Autodesk Fusion 360 part; units mm, degrees
note: some values were not read from the file. Chosen so that the rebuilt part matches the saved one: a direction. Set by a fixed rule: which sketch regions a step uses; which face or edge a step refers to.
(part 6 of 6)
sketch "Sketch34" plane through (0, 0, 0) normal (0, 1, 0) x (1, 0, 0)
  line L0 (0, 0) -> (0, -96.5685)
  line L1 (0, -96.5685) -> (160, -96.5685)
  line L2 (200, -56.5685) -> (200, 0)
  line L3 (200, 0) -> (196, 0)
  arc A0 (160, -96.5685) -> (200, -56.5685) centre (160, -56.5685) ccw
  line L4 (0, 0) -> (0, -88.5685)
  line L5 (0, -88.5685) -> (164, -88.5685)
  line L6 (196, -56.5685) -> (196, 4)
  arc A1 (164, -88.5685) -> (196, -56.5685) centre (164, -56.5685) ccw
  line L7 (196, -56.5685) -> (200, -56.5685)
  line L8 (0, -88.5685) -> (0, -96.5685)
  line L9 (0, 0) -> (0, -83.5685)
  line L10 (0, -83.5685) -> (164, -83.5685)
  line L11 (191, -56.5685) -> (191, -24.5685)
  arc A2 (164, -83.5685) -> (191, -56.5685) centre (164, -56.5685) ccw
  line L12 (0, 0) -> (0, -75.5685)
  line L13 (0, -75.5685) -> (168, -75.5685)
  line L14 (187, -56.5685) -> (187, 0)
  arc A3 (168, -75.5685) -> (187, -56.5685) centre (168, -56.5685) ccw
  line L15 (196, -56.5685) -> (196, -56.3185)
  line L16 (196, -56.5685) -> (196, -56.8185)
  line L17 (196, 0) -> (256, 0) construction
  line L18 (200, 0) -> (143.4315, -56.5685)
  line L19 (200, 0) -> (260, 0) construction
  line L20 (143.4315, -56.5685) -> (187, -56.5685)
  line L21 (187, -56.5685) -> (226.5075, -50.3112)
  line L22 (187, -56.5685) -> (217.0736, -56.5685) construction
  point P0 (200, -96.5685)
  point P1 (196, -88.5685)
  point P2 (191, -83.5685)
  point P3 (187, -75.5685)
  dimension "d479" = 96.5685
  dimension "d480" = 200
  dimension "d481" = 96.5685
  dimension "d482" = 4
  dimension "d483" = 40
  dimension "d484" = 88.5685
  dimension "d485" = 196
  dimension "d486" = 92.5685
  dimension "d487" = 32
  dimension "d488" = 83.5685
  dimension "d489" = 191
  dimension "d490" = 59
  dimension "d491" = 27
  dimension "d492" = 75.5685
  dimension "d493" = 187
  dimension "d494" = 75.5685
  dimension "d495" = 19
  dimension "d496" = 0.25
  dimension "d498" = 0.25
  dimension "d502" = 135
  dimension "d503" = 80
  dimension "d504" = 43.5685
  dimension "d505" = 40
  dimension "d506" = 9
  constraint coincident L0.start L4.start
  constraint vertical L0
  constraint perpendicular L0 L1
  constraint perpendicular L1 L2
  constraint perpendicular L2 L3
  constraint coincident P0 L1
  constraint coincident P0 L2
  constraint tangent L1 A0
  constraint tangent L2 A0
  constraint parallel L0 L4
  constraint perpendicular L4 L5
  constraint perpendicular L5 L6
  constraint coincident P1 L6
  constraint coincident P1 L5
  constraint tangent L6 A1
  constraint tangent L5 A1
  constraint perpendicular L5 L9
  constraint perpendicular L9 L10
  constraint perpendicular L10 L11
  constraint coincident P2 L10
  constraint coincident P2 L11
  constraint tangent L10 A2
  constraint tangent L11 A2
  constraint parallel L4 L12
  constraint perpendicular L12 L13
  constraint perpendicular L13 L14
  constraint coincident P3 L14
  constraint coincident P3 L13
  constraint tangent L14 A3
  constraint tangent L13 A3
  constraint perpendicular L7 L15
  constraint perpendicular L7 L16
  constraint horizontal L17
  constraint horizontal L19
  constraint horizontal L20
  constraint horizontal L22
  measures "d479" distance of L0.start L0.end
  measures "d480" distance of L0.end P0
  measures "d481" distance of P0 L2.end
  measures "d482" distance of L2.end L3.end
  measures "d483" radius of A0
  measures "d484" distance of L0.start L4.end
  measures "d485" distance of L4.end P1
  measures "d486" distance of P1 L6.end
  measures "d487" radius of A1
  measures "d488" distance of L0.start L9.end
  measures "d489" distance of L9.end P2
  measures "d490" distance of P2 L11.end
  measures "d491" radius of A2
  measures "d492" distance of L0.start L12.end
  measures "d493" distance of L12.end P3
  measures "d494" distance of P3 L14.end
  measures "d495" radius of A3
  measures "d496" distance of L6.start L15.end
  measures "d498" distance of L6.start L16.end
  measures "d502" angle of L18 L19
  measures "d503" distance of L2.end L18.end
  measures "d504" distance of L18.end L14.start
  measures "d505" distance of L14.start L21.end
  measures "d506" angle of L21 L22
extrude "Extrude51" add sketch "Sketch34" along normal blind 4 from surface at 4 separate body contours L0 L4 L9 L10 L11 A2 L13 A3 L21 | L0 L1 A0 L5 A1 L7 L8 L16 makes body 14 at (110.6667, 4, 78.2352) makes body 15 at (108, 4, 91.2352)
sketch "rail top 1" plane through (0, 8, 0) normal (0, 1, 0) x (-1, 0, 0)
  line L0 (-164, 88.5685) -> (0, 88.5685)
  line L1 (0, 88.5685) -> (0, 96.5685)
  line L2 (0, 96.5685) -> (-160, 96.5685)
  arc A0 (-160, 96.5685) -> (-200, 56.5685) centre (-160, 56.5685) ccw
  line L3 (-200, 56.5685) -> (-196, 56.5685)
  arc A1 (-164, 88.5685) -> (-196, 56.5685) centre (-164, 56.5685) ccw
  line L4 (0, 96.5685) -> (-8, 96.5685)
  line L5 (-8, 96.5685) -> (-8, 92.5685)
  line L6 (-10, 90.5685) -> (-6, 90.5685)
  line L7 (-6, 90.5685) -> (-6, 94.5685)
  line L8 (-6, 94.5685) -> (-10, 94.5685)
  line L9 (-10, 94.5685) -> (-10, 90.5685)
  line L10 (-10, 90.5685) -> (-6, 94.5685) construction
  line L11 (-6, 90.5685) -> (-10, 94.5685) construction
  point P0 (-8, 92.5685)
  dimension "d513" = 8
  dimension "d514" = 4
  dimension "d515" = 4
  dimension "d516" = 4
  constraint coincident L1.end L2.start
  constraint perpendicular L1 L4
  constraint perpendicular L4 L5
  constraint horizontal L6
  constraint perpendicular L6 L7
  constraint parallel L6 L8
  constraint parallel L7 L9
  constraint coincident L10 P0
  constraint coincident L11 P0
  constraint coincident P0 L5.end
  measures "d513" distance of L1.end L4.end
  measures "d514" distance of L4.end P0
  measures "d515" distance of L7.end L8.end
  measures "d516" distance of L6.end L7.end
extrude "Extrude53" cut sketch "rail top 1" against normal blind 8 contours L6 L7 L8 L9 bodies 2 15
pattern_linear "R-Pattern16" count 3 spacing 72 along (1, 0, 0) of "Extrude53"
sketch "rail bottom 1" plane through (0, 8, 0) normal (0, 1, 0) x (-1, 0, 0)
  line L0 (0, 75.5685) -> (0, 83.5685)
  line L1 (0, 83.5685) -> (-164, 83.5685)
  arc A0 (-164, 83.5685) -> (-191, 56.5685) centre (-164, 56.5685) ccw
  line L2 (-191, 55.935) -> (-187, 56.5685)
  arc A1 (-168, 75.5685) -> (-187, 56.5685) centre (-168, 56.5685) ccw
  line L3 (-168, 75.5685) -> (0, 75.5685)
  line L4 (0, 0) -> (0, 79.5685)
  line L5 (0, 79.5685) -> (-8, 79.5685)
  line L6 (-10, 77.5685) -> (-6, 77.5685)
  line L7 (-6, 77.5685) -> (-6, 81.5685)
  line L8 (-6, 81.5685) -> (-10, 81.5685)
  line L9 (-10, 81.5685) -> (-10, 77.5685)
  line L10 (-10, 77.5685) -> (-6, 81.5685) construction
  line L11 (-6, 77.5685) -> (-10, 81.5685) construction
  line L12 (-191, 56.5685) -> (-191, 55.935)
  point P0 (-8, 79.5685)
  dimension "d523" = 79.5685
  dimension "d524" = 8
  dimension "d525" = 4
  dimension "d526" = 4
  constraint coincident L4.start origin
  constraint midpoint L0 L4.end
  constraint perpendicular L0 L5
  constraint horizontal L6
  constraint perpendicular L6 L7
  constraint parallel L6 L8
  constraint parallel L7 L9
  constraint coincident L10 P0
  constraint coincident L11 P0
  constraint coincident P0 L5.end
  measures "d523" distance of L4.start L4.end
  measures "d524" distance of L4.end P0
  measures "d525" distance of L7.end L8.end
  measures "d526" distance of L6.end L7.end
extrude "Extrude54" cut sketch "rail bottom 1" against normal blind 8 contours L6 L7 L8 L9 bodies 2 14
pattern_linear "R-Pattern17" count 3 spacing 72 along (1, 0, 0) of "Extrude54"
sketch "fingur top rail" plane through (0, 0, 0) normal (-1, 0, 0) x (0, -1, 0)
  line L0 (-4, 88.5685) -> (-4, 96.5685)
  line L1 (-4, 96.5685) -> (-8, 96.5685)
  line L2 (-8, 96.5685) -> (-8, 88.5685)
  line L3 (-8, 88.5685) -> (-4, 88.5685)
  line L4 (-8, 96.5685) -> (-4, 96.5685)
  line L5 (-4, 96.5685) -> (-4, 93.9019)
  line L6 (-4, 93.9019) -> (-8, 93.9019)
  line L7 (-8, 93.9019) -> (-8, 96.5685)
  dimension "d533" = 2.6667
  constraint horizontal L4
  constraint vertical L5
  constraint horizontal L6
  constraint vertical L7
  constraint coincident L0 L5.end
  constraint coincident L1.end L2.start
  measures "d533" distance of L0.end L5.end
extrude "Extrude55" cut sketch "fingur top rail" against normal blind 4 contours L0 L1 L2 L4 L5 L6 L7 bodies 15
pattern_linear "R-Pattern18" count 2 spacing 5.3333 along (0, 0, -1) of "Extrude55"
sketch "fingur bottom rail " plane through (0, 0, 0) normal (-1, 0, 0) x (0, -1, 0)
  line L0 (-4, 75.5685) -> (-4, 83.5685)
  line L1 (-4, 83.5685) -> (-8, 83.5685)
  line L2 (-8, 83.5685) -> (-8, 75.5685)
  line L3 (-8, 75.5685) -> (-4, 75.5685)
  line L4 (-4, 83.5685) -> (-8, 83.5685)
  line L5 (-8, 83.5685) -> (-8, 80.9019)
  line L6 (-8, 80.9019) -> (-4, 80.9019)
  line L7 (-4, 80.9019) -> (-4, 83.5685)
  dimension "d540" = 2.6667
  constraint horizontal L4
  constraint vertical L5
  constraint horizontal L6
  constraint vertical L7
  constraint coincident L2 L5.end
  constraint coincident L0.end L1.start
  measures "d540" distance of L1.end L5.end
extrude "Extrude56" cut sketch "fingur bottom rail " against normal blind 4 contours L0 L1 L2 L4 L5 L6 L7 bodies 14
pattern_linear "R-Pattern19" count 2 spacing 5.3333 along (0, 0, -1) of "Extrude56"
extrude "Extrude52" add 2 faces at (162, 8, 78.9019) (159.3333, 8, 91.9019) along direction (0, -1, 0) blind 4 separate body start surface through (136, 96, 13) normal (0, -1, 0) on bodies 14 15 makes body 16 at (159.3333, 96, 91.9019) makes body 17 at (162, 96, 78.9019)
pattern_linear "R-Pattern20" count 2 spacing 92 along (0, 1, 0) of "Extrude53", "R-Pattern16", "Extrude54", "R-Pattern17"
extrude "Extrude57" cut sketch "rail bottom 1" along normal through all contours L6 L7 L8 L9 bodies 3
pattern_linear "R-Pattern21" count 3 spacing 72 along (1, 0, 0) of "Extrude57"
extrude "Extrude58" cut sketch "rail top 1" along normal through all contours L6 L7 L8 L9 bodies 3
pattern_linear "R-Pattern22" count 3 spacing 72 along (1, 0, 0) of "Extrude58"
sketch "flex sc" plane through (0, 0, 0) normal (0, 0, 1) x (1, 0, 0)
  line L0 (0, 0) -> (250, 0)
  line L1 (250, 0) -> (468.8319, 0)
  line L2 (468.8319, 0) -> (468.8319, 92)
  line L3 (468.8319, 92) -> (250, 92)
  line L4 (250, 92) -> (250, 0)
  dimension "d574" = 250
  dimension "d575" = 218.8319
  dimension "d576" = 92
  constraint coincident L0.start origin
  constraint horizontal L0
  constraint horizontal L1
  constraint vertical L2
  constraint horizontal L3
  constraint vertical L4
  measures "d574" distance of L0.start L0.end
  measures "d575" distance of L0.end L1.end
  measures "d576" distance of L0.end L3.end
extrude "Extrude60" add sketch "flex sc" along normal blind 4 separate body makes body 18
sketch "pinni sc" plane through (0, 0, 0) normal (0, 0, 1) x (1, 0, 0)
  line L0 (0, -20) -> (8, -20)
  line L1 (8, -20) -> (8, -24)
  line L2 (8, -24) -> (0, -24)
  line L3 (0, -24) -> (0, -20)
  dimension "d579" = 8
  dimension "d580" = 4
  constraint horizontal L0
  constraint vertical L1
  constraint horizontal L2
  constraint vertical L3
  measures "d579" distance of L0.start L0.end
  measures "d580" distance of L0.start L2.end
extrude "Extrude61" add sketch "pinni sc" along normal blind 4 separate body makes body 19
pattern_linear "R-Pattern23" count 14 spacing 9 along (1, 0, 0) of bodies 19 makes body 20 at (11.6667, -20, 2.6667) makes body 21 at (20.6667, -20, 2.6667) makes body 22 at (29.6667, -20, 2.6667) makes body 23 at (38.6667, -20, 2.6667) makes body 24 at (47.6667, -20, 2.6667) makes body 25 at (56.6667, -20, 2.6667) makes body 26 at (65.6667, -20, 2.6667) makes body 27 at (74.6667, -20, 2.6667) makes body 28 at (83.6667, -20, 2.6667) makes body 29 at (92.6667, -20, 2.6667) makes body 30 at (101.6667, -20, 2.6667) makes body 31 at (110.6667, -20, 2.6667) makes body 32 at (119.6667, -20, 2.6667)
combine "Combine13" operation cut target body 2 tool bodies 6 keep tools
combine "Combine14" operation cut target body 3 tool bodies 6 keep tools
combine "Combine15" operation cut target body 2 tool bodies 13 12 11 10 9 keep tools
combine "Combine16" operation cut target body 3 tool bodies 13 12 11 10 9 keep tools
combine "Combine17" operation cut target body 4 tool bodies 15 14 16 17 keep tools
sketch "Sketch43" plane through (0, 0, 4) normal (0, 0, 1) x (-1, 0, 0)
  line L0 (-250, -92) -> (-250, 0)
  line L1 (-250, 0) -> (-468.8319, 0)
  line L2 (-468.8319, 0) -> (-468.8319, -92)
  line L3 (-468.8319, -92) -> (-250, -92)
  line L4 (-250, 0) -> (-258, 0)
  line L5 (-258, 0) -> (-258, -92)
  line L6 (-258, -92) -> (-250, -92)
  line L7 (-250, -92) -> (-250, 0)
  line L8 (-250, 0) -> (-252, 0)
  line L9 (-252, 0) -> (-252, -92)
  line L10 (-252, -92) -> (-250, -92)
  line L11 (-250, -92) -> (-250, 0)
  line L12 (-250, 0) -> (-256, 0)
  line L13 (-256, 0) -> (-256, -92)
  line L14 (-256, -92) -> (-250, -92)
  line L15 (-250, -92) -> (-250, 0)
  line L16 (-252, -4) -> (-256, -4)
  line L17 (-256, -4) -> (-256, -88)
  line L18 (-256, -88) -> (-252, -88)
  line L19 (-252, -88) -> (-252, -4)
  dimension "d594" = 8
  dimension "d625" = 2
  dimension "d626" = 92
  dimension "d627" = 6
  dimension "d628" = 92
  dimension "d629" = 4
  dimension "d630" = 84
  constraint horizontal L4
  constraint vertical L5
  constraint horizontal L6
  constraint vertical L7
  constraint coincident L3 L5.end
  constraint coincident L0.end L1.start
  constraint horizontal L8
  constraint vertical L9
  constraint horizontal L10
  constraint vertical L11
  constraint horizontal L12
  constraint vertical L13
  constraint horizontal L14
  constraint vertical L15
  constraint horizontal L16
  constraint vertical L17
  constraint horizontal L18
  constraint vertical L19
  constraint coincident L13 L17.end
  constraint coincident L9 L16.start
  measures "d594" distance of L5 L7
  measures "d625" distance of L0.end L8.end
  measures "d626" distance of L0.end L0.start
  measures "d627" distance of L0.end L12.end
  measures "d628" distance of L0.end L0.start
  measures "d629" distance of L4 L16
  measures "d630" distance of L16 L18
extrude "Extrude63" add sketch "Sketch43" along normal blind 12 from surface at -4 separate body contours L9 L13 L16 L17 L18 L19 makes body 33
sketch "Sketch44" plane through (0, 0, 0) normal (0, 0, -1) x (1, 0, 0)
  line L0 (256, -88) -> (252, -88)
  line L1 (252, -88) -> (252, -81.3333)
  line L2 (252, -81.3333) -> (256, -81.3333)
  line L3 (256, -81.3333) -> (256, -88)
  line L4 (252, -4) -> (252, -88)
  line L5 (252, -88) -> (256, -88)
  line L6 (256, -88) -> (256, -4)
  line L7 (256, -4) -> (252, -4)
  dimension "d613" = 6.6667
  constraint horizontal L0
  constraint vertical L1
  constraint horizontal L2
  constraint vertical L3
  measures "d613" distance of L0 L2
sketch "Sketch45" plane through (0, 0, 4) normal (0, 0, 1) x (-1, 0, 0)
  line L0 (-250, -92) -> (-250, 0)
  line L1 (-250, 0) -> (-468.8319, 0)
  line L2 (-468.8319, 0) -> (-468.8319, -92)
  line L3 (-468.8319, -92) -> (-250, -92)
  line L4 (-250, 0) -> (-252, 0)
  line L5 (-252, 0) -> (-252, -4)
  line L6 (-252, -4) -> (-256, -4)
  line L7 (-256, -4) -> (-256, -10.6667)
  line L8 (-256, -10.6667) -> (-252, -10.6667)
  line L9 (-252, -10.6667) -> (-252, -4)
  dimension "d615" = 2
  dimension "d616" = 4
  dimension "d617" = 4
  dimension "d618" = 6.6667
  constraint coincident L0.end L1.start
  constraint perpendicular L0 L4
  constraint perpendicular L4 L5
  constraint horizontal L6
  constraint vertical L7
  constraint horizontal L8
  constraint vertical L9
  measures "d615" distance of L0.end L4.end
  measures "d616" distance of L4.end L5.end
  measures "d617" distance of L5.end L6.end
  measures "d618" distance of L5.end L8.end
extrude "Extrude64" cut sketch "Sketch45" against normal blind 4 contours L6 L7 L8 L9 bodies 18
pattern_linear "R-Pattern25" count 7 spacing 12.8889 along (0, 1, 0) of "Extrude64"
combine "Combine18" operation cut target body 33 tool bodies 18 keep tools
sketch "Sketch46" plane through (0, 0, 4) normal (0, 0, 1) x (-1, 0, 0)
  line L0 (-256, -81.3333) -> (-252, -81.3333)
  line L1 (-252, -81.3333) -> (-252, -88)
  line L2 (-252, -88) -> (-256, -88)
  line L3 (-256, -88) -> (-256, -81.3333)
  line L4 (-256, -68.4444) -> (-252, -68.4444)
  line L5 (-252, -68.4444) -> (-252, -75.1111)
  line L6 (-252, -75.1111) -> (-256, -75.1111)
  line L7 (-256, -75.1111) -> (-256, -68.4444)
  line L8 (-256, -55.5556) -> (-252, -55.5556)
  line L9 (-252, -55.5556) -> (-252, -62.2222)
  line L10 (-252, -62.2222) -> (-256, -62.2222)
  line L11 (-256, -62.2222) -> (-256, -55.5556)
  line L12 (-256, -42.6667) -> (-252, -42.6667)
  line L13 (-252, -42.6667) -> (-252, -49.3333)
  line L14 (-252, -49.3333) -> (-256, -49.3333)
  line L15 (-256, -49.3333) -> (-256, -42.6667)
  line L16 (-256, -29.7778) -> (-252, -29.7778)
  line L17 (-252, -29.7778) -> (-252, -36.4444)
  line L18 (-252, -36.4444) -> (-256, -36.4444)
  line L19 (-256, -36.4444) -> (-256, -29.7778)
  line L20 (-256, -16.8889) -> (-252, -16.8889)
  line L21 (-252, -16.8889) -> (-252, -23.5556)
  line L22 (-252, -23.5556) -> (-256, -23.5556)
  line L23 (-256, -23.5556) -> (-256, -16.8889)
  line L24 (-256, -4) -> (-252, -4)
  line L25 (-252, -4) -> (-252, -10.6667)
  line L26 (-252, -10.6667) -> (-256, -10.6667)
  line L27 (-256, -10.6667) -> (-256, -4)
  line L28 (-250, -92) -> (-250, 0)
  line L29 (-250, 0) -> (-468.8319, 0)
  line L30 (-468.8319, 0) -> (-468.8319, -92)
  line L31 (-468.8319, -92) -> (-250, -92)
  line L32 (-250, 0) -> (-258, 0)
  line L33 (-258, 0) -> (-258, -92)
  line L34 (-258, -92) -> (-250, -92)
  line L35 (-250, -92) -> (-250, 0)
  line L36 (-258, 0) -> (-259, 0)
  line L37 (-259, 0) -> (-259, -61.3333)
  line L38 (-259, -61.3333) -> (-258, -61.3333)
  line L39 (-258, -61.3333) -> (-258, 0)
  line L40 (-250, -92) -> (-260, -92)
  line L41 (-260, -92) -> (-261, -92)
  line L42 (-261, -92) -> (-261, -30.6667)
  line L43 (-261, -30.6667) -> (-260, -30.6667)
  line L44 (-260, -30.6667) -> (-260, -92)
  dimension "d632" = 8
  dimension "d634" = 1
  dimension "d635" = 61.3333
  dimension "d636" = 10
  dimension "d637" = 1
  dimension "d638" = 61.3333
  constraint horizontal L32
  constraint vertical L33
  constraint horizontal L34
  constraint vertical L35
  constraint coincident L31 L33.end
  constraint coincident L28.end L29.start
  constraint horizontal L36
  constraint vertical L37
  constraint horizontal L38
  constraint vertical L39
  constraint perpendicular L33 L40
  constraint horizontal L41
  constraint vertical L42
  constraint horizontal L43
  constraint vertical L44
  measures "d632" distance of L33.end L28.start
  measures "d634" distance of L32.end L36.end
  measures "d635" distance of L32.end L38.end
  measures "d636" distance of L28.start L40.end
  measures "d637" distance of L40.end L41.end
  measures "d638" distance of L40.end L43.end
extrude "Extrude65" cut sketch "Sketch46" against normal blind 4 contours L29 L33 L36 L37 L38 L39 bodies 18
extrude "Extrude66" cut sketch "Sketch46" against normal blind 4 contours L31 L41 L42 L43 L44 bodies 18
pattern_linear "R-Pattern26" count 53 spacing 4 along (1, 0, 0) of "Extrude65"
pattern_linear "R-Pattern27" count 52 spacing 4 along (1, 0, 0) of "Extrude66"
copy_body "Body->Comp1" bodies 1 removing the originals makes body 34 in component "botnplata_body"
copy_body "Body->Comp2" bodies 2 removing the originals makes body 35 in component "hliðarplata body"
copy_body "Body->Comp3" bodies 3 removing the originals makes body 36 in component "hliðarplata 2 body"
copy_body "Body->Comp4" bodies 4 removing the originals makes body 37 in component "bakplata"
copy_body "Body->Comp5" bodies 5 removing the originals makes body 38 in component "fremriplata"
copy_body "Body->Comp6" bodies 6 removing the originals makes body 39 in component "milliplata"
copy_body "Body->Comp7" bodies 7 removing the originals makes body 40 in component "rail1"
copy_body "Body->Comp8" bodies 8 removing the originals makes body 41 in component "rail2"
copy_body "Body->Comp9" bodies 9 removing the originals makes body 42 in component "guide1"
copy_body "Body->Comp10" bodies 10 removing the originals makes body 43 in component "guide2"
copy_body "Body->Comp11" bodies 11 removing the originals makes body 44 in component "guide3"
copy_body "Body->Comp12" bodies 12 removing the originals makes body 45 in component "guide4"
copy_body "Body->Comp13" bodies 13 removing the originals makes body 46 in component "guide5"
copy_body "Body->Comp14" bodies 14 removing the originals makes body 47 in component "guide top 1"
copy_body "Body->Comp15" bodies 15 removing the originals makes body 48 in component "guide bottom 1"
copy_body "Body->Comp16" bodies 17 removing the originals makes body 49 in component "guide bottom 2"
copy_body "Body->Comp17" bodies 16 removing the originals makes body 50 in component "guide top 2"
copy_body "Body->Comp18" bodies 18 removing the originals makes body 51 in component "flex plate"
copy_body "Body->Comp19" bodies 19 removing the originals makes body 52 in component "p1"
copy_body "Body->Comp20" bodies 20 removing the originals makes body 53 in component "p2"
copy_body "Body->Comp21" bodies 21 removing the originals makes body 54 in component "p3"
copy_body "Body->Comp22" bodies 22 removing the originals makes body 55 in component "p4"
copy_body "Body->Comp23" bodies 23 removing the originals makes body 56 in component "p6"
copy_body "Body->Comp24" bodies 24 removing the originals makes body 57 in component "p7"
copy_body "Body->Comp25" bodies 25 removing the originals makes body 58 in component "p8"
copy_body "Body->Comp26" bodies 26 removing the originals makes body 59 in component "p9"
copy_body "Body->Comp27" bodies 27 removing the originals makes body 60 in component "p10"
copy_body "Body->Comp28" bodies 28 removing the originals makes body 61 in component "p11"
copy_body "Body->Comp29" bodies 29 removing the originals makes body 62 in component "p12"
copy_body "Body->Comp30" bodies 30 removing the originals makes body 63 in component "p13"
copy_body "Body->Comp31" bodies 31 removing the originals makes body 64 in component "p14"
copy_body "Body->Comp32" bodies 32 removing the originals makes body 65 in component "p15"
copy_body "Body->Comp33" bodies 33 removing the originals makes body 66 in component "stoppari"
extrude "Extrude1'" cut sketch "hola" along normal blind 100 bodies 36 in component "hliðarplata 2 body"
component "Box" placed x (1, 0, 0) y (0, 1, 0) z (0, 0, 1) at (0, 0, 0)
component "stoppari" placed x (1, 0, 0) y (0, 1, 0) z (0, 0, 1) at (0, 0, 0) in component "Box"
component "guide bottom 2" placed x (1, 0, 0) y (0, 1, 0) z (0, 0, 1) at (0, 0, 0) in component "Box"
component "p3" placed x (1, 0, 0) y (0, 1, 0) z (0, 0, 1) at (0, 0, 0) in component "Box"
component "p6" placed x (1, 0, 0) y (0, 1, 0) z (0, 0, 1) at (0, 0, 0) in component "Box"
component "guide top 2" placed x (1, 0, 0) y (0, 1, 0) z (0, 0, 1) at (0, 0, 0) in component "Box"
component "flex plate" placed x (1, 0, 0) y (0, 1, 0) z (0, 0, 1) at (0, 0, 0) in component "Box"
component "p1" placed x (1, 0, 0) y (0, 1, 0) z (0, 0, 1) at (0, 0, 0) in component "Box"
component "p2" placed x (1, 0, 0) y (0, 1, 0) z (0, 0, 1) at (0, 0, 0) in component "Box"
component "p4" placed x (1, 0, 0) y (0, 1, 0) z (0, 0, 1) at (0, 0, 0) in component "Box"
component "p7" placed x (1, 0, 0) y (0, 1, 0) z (0, 0, 1) at (0, 0, 0) in component "Box"
component "p8" placed x (1, 0, 0) y (0, 1, 0) z (0, 0, 1) at (0, 0, 0) in component "Box"
component "p9" placed x (1, 0, 0) y (0, 1, 0) z (0, 0, 1) at (0, 0, 0) in component "Box"
component "p10" placed x (1, 0, 0) y (0, 1, 0) z (0, 0, 1) at (0, 0, 0) in component "Box"
component "p11" placed x (1, 0, 0) y (0, 1, 0) z (0, 0, 1) at (0, 0, 0) in component "Box"
component "botnplata_body" placed x (1, 0, 0) y (0, 1, 0) z (0, 0, 1) at (0, 0, 0) in component "Box"
component "milliplata" placed x (1, 0, 0) y (0, 1, 0) z (0, 0, 1) at (0, 0, 0) in component "Box"
component "rail2" placed x (1, 0, 0) y (0, 1, 0) z (0, 0, 1) at (0, 0, 0) in component "Box"
component "guide1" placed x (1, 0, 0) y (0, 1, 0) z (0, 0, 1) at (0, 0, 0) in component "Box"
component "guide3" placed x (1, 0, 0) y (0, 1, 0) z (0, 0, 1) at (0, 0, 0) in component "Box"
component "guide5" placed x (1, 0, 0) y (0, 1, 0) z (0, 0, 1) at (0, 0, 0) in component "Box"
component "guide top 1" placed x (1, 0, 0) y (0, 1, 0) z (0, 0, 1) at (0, 0, 0) in component "Box"
component "rail1" placed x (1, 0, 0) y (0, 1, 0) z (0, 0, 1) at (0, 0, 0) in component "Box"
component "guide4" placed x (1, 0, 0) y (0, 1, 0) z (0, 0, 1) at (0, 0, 0) in component "Box"
component "guide2" placed x (1, 0, 0) y (0, 1, 0) z (0, 0, 1) at (0, 0, 0) in component "Box"
component "guide bottom 1" placed x (1, 0, 0) y (0, 1, 0) z (0, 0, 1) at (0, 0, 0) in component "Box"
component "bakplata" placed x (1, 0, 0) y (0, 1, 0) z (0, 0, 1) at (0, 0, 0) in component "Box"
component "hliðarplata 2 body" placed x (1, 0, 0) y (0, 1, 0) z (0, 0, 1) at (0, 0, 0) in component "Box"
component "fremriplata" placed x (1, 0, 0) y (0, 1, 0) z (0, 0, 1) at (0, 0, 0) in component "Box"
component "hliðarplata body" placed x (1, 0, 0) y (0, 1, 0) z (0, 0, 1) at (0, 0, 0) in component "Box"
component "p14" placed x (1, 0, 0) y (0, 1, 0) z (0, 0, 1) at (0, 0, 0) in component "Box"
component "p15" placed x (1, 0, 0) y (0, 1, 0) z (0, 0, 1) at (0, 0, 0) in component "Box"
component "p12" placed x (1, 0, 0) y (0, 1, 0) z (0, 0, 1) at (0, 0, 0) in component "Box"
component "p13" placed x (1, 0, 0) y (0, 1, 0) z (0, 0, 1) at (0, 0, 0) in component "Box"
equation "þykkt_plotu = 4 mm"
equation "lengd = 200 mm"
equation "breidd = 100 mm"
equation "hæð = ( 1 + sqrt(2) ) * radius"
equation "lfingur = 15"
equation "bfingur = 7"
equation "hfingur = 6"
equation "lfingurbreidd = lengd / ( ( lfingur * 2 ) + 1 )"
equation "bfingurbreidd = breidd / ( ( bfingur * 2 ) + 1 )"
equation "hfingurbreidd = hæð / ( ( hfingur * 2 ) + 1 )"
equation "d216 = lengd"
equation "d217 = breidd"
equation "breidd_slider = breidd - ( 2 * þykkt_plotu )"
equation "lengd_slider = lengd - radius + ( radius ) * PI / 2 - þykkt_plotu"
equation "d220 = þykkt_plotu"
equation "d222 = lfingurbreidd"
equation "d223 = lfingurbreidd"
equation "d224 = -þykkt_plotu"
equation "d226 = lfingur"
equation "d228 = ( lengd - ( lfingurbreidd * 3 ) )"
equation "d230 = hæð"
equation "d231 = þykkt_plotu"
equation "d233 = hfingurbreidd"
equation "d235 = -þykkt_plotu"
equation "d237 = hfingur"
equation "d239 = -( hæð - ( hfingurbreidd * 3 ) )"
equation "d241 = hfingurbreidd"
equation "radius = 40 mm"
equation "d244 = radius"
equation "d245 = hfingurbreidd"
equation "d246 = hfingurbreidd"
equation "d247 = -þykkt_plotu"
equation "d249 = hfingur - floor(radius / 2 / hfingurbreidd)"
equation "d251 = hæð - radius - 3 * hfingurbreidd"
equation "d254 = -þykkt_plotu"
equation "d256 = bfingurbreidd"
equation "d257 = bfingurbreidd"
equation "d258 = -þykkt_plotu"
equation "d260 = bfingur"
equation "d262 = -( breidd - 3 * bfingurbreidd )"
equation "d264 = breidd"
equation "d265 = hæð"
equation "d266 = þykkt_plotu"
equation "d268 = bfingurbreidd"
equation "d269 = bfingurbreidd"
equation "d270 = -þykkt_plotu"
equation "d272 = bfingur"
equation "d274 = breidd - 3 * bfingurbreidd"
equation "d276 = hæð - radius"
equation "d277 = -þykkt_plotu"
equation "d280 = þykkt_plotu"
equation "d281 = breidd"
equation "d282 = lengd - 2 * radius / sqrt(2) - þykkt_plotu"
equation "d283 = 2 * þykkt_plotu + 1 mm"
equation "d284 = þykkt_plotu"
equation "milliplata_fingur = floor(lfingur - ( radius + þykkt_plotu ) / lfingurbreidd)"
equation "milliplata_fingur_breidd = ( lengd - radius - þykkt_plotu ) / ( milliplata_fingur * 2 + 1 )"
equation "d288 = milliplata_fingur_breidd"
equation "d289 = -þykkt_plotu"
equation "d291 = milliplata_fingur"
equation "d293 = ( lengd - radius - þykkt_plotu - ( 3 * milliplata_fingur ) * 1 mm )"
equation "d295 = milliplata_fingur_breidd"
equation "d296 = -þykkt_plotu"
equation "d298 = milliplata_fingur"
equation "d300 = ( lengd - radius - þykkt_plotu - ( 3 * milliplata_fingur ) * 1 mm )"
equation "d429 = lengd - þykkt_plotu"
equation "d430 = lengd"
equation "d431 = lengd"
equation "d433 = 2 * radius"
equation "d434 = ( sqrt(2) * radius - 3 * þykkt_plotu ) * 2 - 2 mm"
equation "d435 = 2 * radius - þykkt_plotu * 3"
equation "d436 = 2 * ( sqrt(2) * radius - 3 * þykkt_plotu )"
equation "d437 = þykkt_plotu"
equation "d438 = þykkt_plotu"
equation "d439 = þykkt_plotu"
equation "d440 = þykkt_plotu"
equation "d443 = -þykkt_plotu"
equation "d445 = lengd - þykkt_plotu * 2"
equation "d446 = þykkt_plotu * 2"
equation "d447 = þykkt_plotu"
equation "d448 = þykkt_plotu"
equation "d460 = sqrt(2) * radius - 3 * þykkt_plotu - 1 mm"
equation "d461 = ( 90 / 5 ) * 1 deg"
equation "d462 = þykkt_plotu"
equation "d463 = breidd"
equation "d466 = ( sqrt(2) * radius - 1 mm - 3 * þykkt_plotu ) * PI / 10"
equation "d469 = 2 * ( sqrt(2) * radius - 1 mm - 3 * þykkt_plotu ) * sin(( 90 / 10 ) * 1 deg) / 3"
equation "d470 = -þykkt_plotu"
equation "d474 = -2 * ( sqrt(2) * radius - 3 * þykkt_plotu ) * sin(( 90 / 5 ) * 1 deg) / 3"
equation "d476 = -breidd + þykkt_plotu"
equation "d477 = þykkt_plotu"
equation "d479 = hæð"
equation "d480 = lengd"
equation "d481 = hæð"
equation "d482 = þykkt_plotu"
equation "d483 = radius"
equation "d484 = hæð - þykkt_plotu * 2"
equation "d485 = lengd - þykkt_plotu"
equation "d486 = hæð - þykkt_plotu"
equation "d487 = radius - þykkt_plotu * 2"
equation "d488 = hæð - 3 * þykkt_plotu - 1 mm"
equation "d489 = lengd - 2 * þykkt_plotu - 1 mm"
equation "d491 = radius - 3 * þykkt_plotu - 1 mm"
equation "d492 = hæð - 3 * þykkt_plotu - 1 mm - þykkt_plotu * 2"
equation "d493 = lengd - 2 * þykkt_plotu - þykkt_plotu - 1 mm"
equation "d494 = hæð - 5 * þykkt_plotu - 1 mm"
equation "d495 = radius - 5 * þykkt_plotu - 1 mm"
equation "d503 = radius * 2"
equation "d504 = sqrt(2) * radius - 3 * þykkt_plotu - 1 mm"
equation "d505 = radius"
equation "d506 = ( 18 / 2 ) * 1 deg"
equation "d507 = þykkt_plotu"
equation "d508 = þykkt_plotu"
equation "d511 = -þykkt_plotu"
equation "d513 = þykkt_plotu * 2"
equation "d514 = þykkt_plotu"
equation "d515 = þykkt_plotu"
equation "d516 = þykkt_plotu"
equation "d517 = -2 * þykkt_plotu"
equation "d521 = lengd - radius - þykkt_plotu * 4"
equation "d523 = hæð - þykkt_plotu * 4 - 1 mm"
equation "d524 = þykkt_plotu * 2"
equation "d525 = þykkt_plotu"
equation "d526 = þykkt_plotu"
equation "d527 = -2 * þykkt_plotu"
equation "d531 = lengd - radius - 4 * þykkt_plotu"
equation "d533 = 2 / 3 * þykkt_plotu"
equation "d534 = -þykkt_plotu"
equation "d538 = 2 * þykkt_plotu - 2 / 3 * þykkt_plotu"
equation "d540 = 2 / 3 * þykkt_plotu"
equation "d541 = -þykkt_plotu"
equation "d545 = -2 * þykkt_plotu + 2 / 3 * þykkt_plotu"
equation "d549 = breidd - 2 * þykkt_plotu"
equation "d554 = lengd - radius - 4 * þykkt_plotu"
equation "d559 = lengd - radius - 4 * þykkt_plotu"
equation "d561 = breidd"
equation "d574 = lengd + 50 mm"
equation "d575 = lengd - radius + ( radius ) * PI / 2 - þykkt_plotu"
equation "d576 = breidd - 2 * þykkt_plotu"
equation "d577 = þykkt_plotu"
equation "d579 = þykkt_plotu * 2"
equation "d580 = þykkt_plotu"
equation "d581 = þykkt_plotu"
equation "d583 = 8 + 6"
equation "d585 = 2 * þykkt_plotu + 1 mm"
equation "d587 = lengd"
equation "d588 = hæð - radius - þykkt_plotu * 2"
equation "d589 = þykkt_plotu"
equation "d590 = hæð - þykkt_plotu * 2 - radius"
equation "d591 = þykkt_plotu"
equation "d592 = hæð"
equation "d593 = hæð"
equation "d594 = þykkt_plotu * 2"
equation "d610 = -þykkt_plotu"
equation "d611 = þykkt_plotu * 3"
equation "d613 = bfingurbreidd"
equation "d615 = þykkt_plotu / 2"
equation "d616 = þykkt_plotu"
equation "d617 = þykkt_plotu"
equation "d618 = bfingurbreidd"
equation "d619 = -þykkt_plotu"
equation "d621 = bfingur"
equation "d623 = breidd - 4 * þykkt_plotu - bfingurbreidd"
equation "d625 = þykkt_plotu / 2"
equation "d626 = breidd - 2 * þykkt_plotu"
equation "d627 = 3 / 2 * þykkt_plotu"
equation "d628 = breidd - 2 * þykkt_plotu"
equation "d629 = þykkt_plotu"
equation "d630 = breidd - 4 * þykkt_plotu"
equation "kerf = 0.1 mm"
equation "d632 = 2 * þykkt_plotu"
equation "fjöldilínaslider = floor(( lengd_slider - 2 * þykkt_plotu + 3 mm ) / ( 4 mm ))"
equation "d635 = breidd_slider / 1.5"
equation "d636 = 2 * þykkt_plotu + 2 mm"
equation "d638 = breidd_slider / 1.5"
equation "d639 = -þykkt_plotu"
equation "d641 = -þykkt_plotu"
equation "d643 = fjöldilínaslider"
equation "d647 = fjöldilínaslider - 1"
equation "d651 = breidd"
named bodies: "botnplata_body", "hliðarplata body", "hliðarplata 2 body", "bakplata", "fremriplata", "milliplata", "rail1", "rail2", "guide1", "guide2", "guide3", "guide4", "guide5", "guide top 1", "guide bottom 1", "guide top 2", "guide bottom 2", "flex plate", "p1", "p2", "p3", "p4", "p6", "p7", "p8", "p9", "p10", "p11", "p12", "p13", "p14", "p15", "stoppari"
